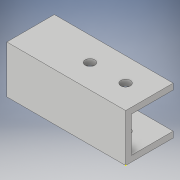
# Autodesk Inventor part: wheel tip connector 1
Saved by Autodesk Inventor 2018 (Build 220112000, 112)
## iProperties
Created: 2019-02-23
Part Number: wheel tip connector 1
Material: Generic
Document SubType Name: Modeling
Designer: s-2513225
Density: 1 g/cm^3
Appearance: Default
Author: s-2513225
Autodesk Inventor part; units mm, degrees
ref_plane "YZ Plane" through (0, 0, 0) normal (1, 0, 0) x (0, 1, 0)
ref_plane "XZ Plane" through (0, 0, 0) normal (0, 1, 0) x (-1, 0, 0)
ref_plane "XY Plane" through (0, 0, 0) normal (0, 0, 1) x (1, 0, 0)
sketch "Sketch1" plane through (0, 0, 0) normal (0, 1, 0) x (-1, 0, 0)
  line L0 (0, 0) -> (63.5, 0)
  line L1 (63.5, 0) -> (63.5, -25.4)
  line L2 (63.5, -25.4) -> (0, -25.4)
  line L3 (0, -25.4) -> (0, 0)
  dimension "d0" = 63.5
  dimension "d1" = 25.4
  constraints: 8 end point, 2 parallel, 1 horizontal, 1 perpendicular
  measures "d0" distance of L1.end L2.end
  measures "d1" distance of L0.end L1.end
extrude "Extrusion1" add sketch "Sketch1" along normal blind 25.4
sketch "Sketch2" plane through (0, 0, 0) normal (1, 0, 0) x (0, 0, -1)
  point P0 (0, 0)
sketch "Sketch3" plane through (0, 0, 0) normal (1, 0, 0) x (0, 0, -1)
  line L0 (25.4, 0) -> (0, 0) projected
  line L1 (25.4, 0) -> (25.4, 25.4) projected
  line L2 (0, 25.4) -> (25.4, 25.4) projected
  line L3 (0, 0) -> (0, 25.4) projected
  line L4 (22.225, 3.175) -> (3.175, 3.175)
  line L5 (3.175, 3.175) -> (3.175, 22.225)
  line L6 (3.175, 22.225) -> (22.225, 22.225)
  line L7 (22.225, 22.225) -> (25.4, 22.225)
  line L8 (25.4, 0) -> (25.4, 25.4) projected
  line L9 (22.225, 3.175) -> (25.4, 3.175)
  line L10 (25.4, 22.225) -> (25.4, 3.175)
  dimension "d4" = 3.175
  constraints: 12 end point, 2 point on line, 1 collinear, 1 parallel, 1 perpendicular, 2 other
  measures "d4" distance between parallel lines of L2 L6
sketch "Sketch4" plane through (0, 25.4, 0) normal (0, 1, 0) x (1, 0, 0)
  line L0 (-63.5, 0) -> (-63.5, 25.4) construction
  line L1 (-63.5, 12.7) -> (0, 12.7) construction
  line L2 (0, 12.7) -> (-12.7, 12.7) construction
  line L3 (-12.7, 12.7) -> (-31.75, 12.7) construction
  circle A0 centre (-31.75, 12.7) radius 2.5797
  circle A1 centre (-12.7, 12.7) radius 2.5797
  point P0 (0, 0)
  dimension "d7" = 12.7
  dimension "d8" = 19.05
  dimension "d9" = 5.1594
  dimension "d10" = 5.1594
  constraints: 6 end point, 2 centre point, 2 coincident, 2 midpoint, 1 horizontal, 1 point on line
  measures "d7" distance of L1.end L2.end
  measures "d8" distance of L2.end L3.end
  measures "d9" diameter of A0
  measures "d10" diameter of A1
extrude "Extrusion3" cut sketch "Sketch4" against normal blind 63.5
extrude "Extrusion4" cut sketch "Sketch3" against normal blind 127 contours L9 L4 L5 L6 L7 L1
body "Solid1"
